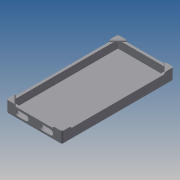
# Autodesk Inventor part: Attempt 3
Saved by Autodesk Inventor 2014 (Build 180170000, 170)
## iProperties
Created: 2014-04-30
Part Number: Attempt 3
Material: Generic
Document SubType Name: Modeling
Designer: 1770749
Density: 1 g/cm^3
Appearance: Default
Author: 1770749
Autodesk Inventor part; units mm, degrees
ref_plane "YZ Plane" through (0, 0, 0) normal (1, 0, 0) x (0, 1, 0)
ref_plane "XZ Plane" through (0, 0, 0) normal (0, 1, 0) x (-1, 0, 0)
ref_plane "XY Plane" through (0, 0, 0) normal (0, 0, 1) x (1, 0, 0)
sketch "Sketch1" plane through (0, 0, 0) normal (0, 0, 1) x (1, 0, 0)
  line L0 (0, 0) -> (59.18, 0)
  line L1 (59.18, 0) -> (59.18, 124.44)
  line L2 (59.18, 124.44) -> (0, 124.44)
  line L3 (0, 124.44) -> (0, 0)
  dimension "d0" = 59.18
  dimension "d1" = 124.44
  constraints: 8 end point, 2 parallel, 1 horizontal, 1 perpendicular
  measures "d0" distance of L2.end L1.end
  measures "d1" distance of L1.end L0.end
sketch "Sketch2" plane through (0, 0, 0) normal (0, 0, 1) x (1, 0, 0)
  line L0 (-3, 127.44) -> (62.18, 127.44)
  line L1 (62.18, 127.44) -> (62.18, -3)
  line L2 (62.18, -3) -> (-3, -3)
  line L3 (-3, -3) -> (-3, 127.44)
  line L4 (59.18, 0) -> (59.18, 124.44) projected
  line L5 (59.18, 124.44) -> (0, 124.44) projected
  line L6 (0, 124.44) -> (0, 0) projected
  line L7 (0, 0) -> (59.18, 0) projected
  dimension "d2" = 3
  dimension "d3" = 3
  dimension "d4" = 3
  dimension "d5" = 3
  constraints: 8 end point, 2 parallel, 1 horizontal, 1 perpendicular
  measures "d2" distance between parallel lines of L1 L4
  measures "d3" distance between parallel lines of L0 L5
  measures "d4" distance between parallel lines of L6 L3
  measures "d5" distance between parallel lines of L2 L7
extrude "Extrusion1" add sketch "Sketch2" against normal blind 12 contours L0 L1 L2 L3 | L7 L6 L5 L4
extrude "Extrusion2" cut sketch "Sketch1" against normal blind 8.97
fillet "Fillet1" radius 2 1 edges at (62.18, 127.44, -6)
fillet "Fillet2" radius 2 1 edges at (-3, 127.44, -6)
fillet "Fillet3" radius 2 2 edges at (62.18, -3, -6) (-3, -3, -6)
fillet "Fillet4" radius 2 8 edges at (61.5942, -2.4142, -12) (29.59, -3, -12) (-2.4142, -2.4142, -12) (-3, 62.22, -12) (-2.4142, 126.8542, -12) (29.59, 127.44, -12) (61.5942, 126.8542, -12) (62.18, 62.22, -12)
sketch "Sketch5" plane through (0, 0, 0) normal (0, 0, 1) x (1, 0, 0)
  arc A0 (-3, -1) -> (-1, -3) centre (-1, -1) ccw projected
  line L0 (60.18, -3) -> (-1, -3) projected
  line L1 (-3, -1) -> (-3, 125.44) projected
  line L2 (-3, 8) -> (8, -3)
  line L3 (-3, 8) -> (12.5563, 8) construction
  line L4 (8, -3) -> (-1, -3)
  line L5 (-3, 8) -> (-3, -1)
  arc A1 (-3, -1) -> (-1, -3) centre (-1, -1) ccw
  line L6 (-1, 127.44) -> (60.18, 127.44) projected
  arc A2 (-1, 127.44) -> (-3, 125.44) centre (-1, 125.44) ccw projected
  line L7 (-3, 116.44) -> (8, 127.44)
  line L8 (-3, 125.44) -> (-3, 116.44)
  line L9 (-1, 127.44) -> (8, 127.44)
  arc A3 (-1, 127.44) -> (-3, 125.44) centre (-1, 125.44) ccw
  line L10 (62.18, 125.44) -> (62.18, -1) projected
  arc A4 (62.18, 125.44) -> (60.18, 127.44) centre (60.18, 125.44) ccw projected
  arc A5 (60.18, -3) -> (62.18, -1) centre (60.18, -1) ccw projected
  line L11 (51.18, 127.44) -> (62.18, 116.44)
  line L12 (51.18, 127.44) -> (60.18, 127.44)
  line L13 (62.18, 125.44) -> (62.18, 116.44)
  arc A6 (62.18, 125.44) -> (60.18, 127.44) centre (60.18, 125.44) ccw
  line L14 (60.18, -3) -> (51.18, -3)
  line L15 (62.18, -1) -> (62.18, 8)
  line L16 (62.18, 8) -> (51.18, -3)
  arc A7 (60.18, -3) -> (62.18, -1) centre (60.18, -1) ccw
  dimension "d18" = 45
  dimension "d21" = 11
  dimension "d22" = 11
  dimension "d23" = 45
  dimension "d26" = 11
  dimension "d27" = 45
  dimension "d28" = 11
  dimension "d29" = 45
  constraints: 26 end point, 10 point on circle, 10 tangent, 8 point on line, 4 centre point, 4 collinear, 3 perpendicular, 1 concentric, 1 equal length, 1 horizontal
  measures "d18" angle of L2 L3
  measures "d21" distance from line of L0 L2.start
  measures "d22" distance from line of L7.start L6
  measures "d23" angle of L1 L7
  measures "d26" distance from line of L6 L11.end
  measures "d27" angle of L10 L11
  measures "d28" distance from line of L14 L15.end
  measures "d29" angle of L10 L16
extrude "Extrusion6" add sketch "Sketch5" along normal blind 2 contours L1 L2 L0 A0 | L1 A2 L6 L7 | L16 L10 A5 L0 | L6 A4 L10 L11
sketch "Sketch6" plane through (-1, -3, -10) normal (0, -1, 0) x (1, 0, 0)
  line L0 (61.18, 0) -> (0, 0) projected
  line L1 (61.18, 0) -> (61.18, 12) projected
  line L2 (49.68, 4.37) -> (40.2, 4.37) construction
  line L3 (49.68, 1.37) -> (40.2, 1.37)
  line L4 (40.2, 7.37) -> (49.68, 7.37)
  arc A0 (49.68, 1.37) -> (49.68, 7.37) centre (49.68, 4.37) ccw
  arc A1 (40.2, 7.37) -> (40.2, 1.37) centre (40.2, 4.37) ccw
  point P0 (1, 10)
  point P1 (44.94, 4.37)
  dimension "d33" = 1.37
  dimension "d35" = 3
  dimension "d36" = 9.48
  dimension "d37" = 8.5
  constraints: 8 end point, 4 point on circle, 4 tangent, 2 centre point, 2 parallel, 1 midpoint
  measures "d33" distance between parallel lines of L0 L3
  measures "d35" distance between parallel lines of L2 L4
  measures "d36" distance of L2.start L2.end
  measures "d37" distance edge to line of A0 L1
extrude "Extrusion7" cut sketch "Sketch6" against normal up to next
sketch "Sketch7" plane through (-1, -3, -10) normal (0, -1, 0) x (1, 0, 0)
  line L0 (49.68, 1.37) -> (40.2, 1.37) projected
  line L1 (61.18, 0) -> (0, 0) projected
  line L2 (0, 0) -> (0, 12) projected
  line L3 (20.98, 4.37) -> (11.5, 4.37) construction
  line L4 (20.98, 1.37) -> (11.5, 1.37)
  line L5 (11.5, 7.37) -> (20.98, 7.37)
  arc A0 (20.98, 1.37) -> (20.98, 7.37) centre (20.98, 4.37) ccw
  arc A1 (11.5, 7.37) -> (11.5, 1.37) centre (11.5, 4.37) ccw
  point P0 (1, 10)
  point P1 (16.24, 4.37)
  dimension "d40" = 1.37
  dimension "d41" = 9.48
  dimension "d42" = 8.5
  dimension "d43" = 3
  constraints: 8 end point, 4 point on circle, 4 tangent, 2 centre point, 2 parallel, 1 midpoint
  measures "d40" distance between parallel lines of L1 L4
  measures "d41" distance of L4.start L4.end
  measures "d42" distance edge to line of A1 L2
  measures "d43" distance between parallel lines of L3 L5
extrude "Extrusion8" cut sketch "Sketch7" against normal up to next
fillet "Fillet5" radius 2 4 edges at (2.5, 121.94, 2) (56.68, 121.94, 2) (2.5, 2.5, 2) (56.68, 2.5, 2)
body "Solid1"
